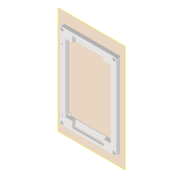
# Autodesk Inventor part: 30_xystage_gp-010b_adapter_multiwellplate
Saved by Autodesk Inventor 2022 (Build 260153000, 153)
## iProperties
Created: 2023-06-03
Part Number: 30_xystage_gp-010b_adapter_multiwellplate
Material: Generisch
Document SubType Name: Modeling
Designer: diederichbenedict
Density: 1 g/cm^3
Appearance: Vorgabe
Author: diederichbenedict
Autodesk Inventor part; units mm, degrees
ref_plane "YZ Plane" through (0, 0, 0) normal (1, 0, 0) x (0, 1, 0)
ref_plane "XZ Plane" through (0, 0, 0) normal (0, 1, 0) x (-1, 0, 0)
ref_plane "XY Plane" through (0, 0, 0) normal (0, 0, 1) x (1, 0, 0)
ref_plane "Arbeitsebene1" through (0, 0, 0) normal (0, 0, 1) x (1, 0, 0)
sketch "Skizze1" plane through (0, 0, 0) normal (0, 0, 1) x (1, 0, 0)
  line L0 (50, 77.5) -> (-50, 77.5) construction
  line L1 (-50, 77.5) -> (-50, -77.5) construction
  line L2 (-50, -77.5) -> (50, -77.5) construction
  line L3 (50, -77.5) -> (50, 77.5) construction
  line L4 (51, 82.5) -> (-51, 82.5)
  line L5 (-55, 78.5) -> (-55, -78.5)
  line L6 (-51, -82.5) -> (51, -82.5)
  line L7 (55, -78.5) -> (55, 78.5)
  circle A0 centre (50, 77.5) radius 1.6
  circle A1 centre (50, -77.5) radius 1.6
  circle A2 centre (-50, -77.5) radius 1.6
  circle A3 centre (-50, 77.5) radius 1.6
  arc A4 (55, 78.5) -> (51, 82.5) centre (51, 78.5) ccw
  arc A5 (51, -82.5) -> (55, -78.5) centre (51, -78.5) ccw
  arc A6 (-55, -78.5) -> (-51, -82.5) centre (-51, -78.5) ccw
  arc A7 (-51, 82.5) -> (-55, 78.5) centre (-51, 78.5) ccw
  line L8 (43, 64.5) -> (43, -64.5)
  line L9 (-43, -64.5) -> (-43, 64.5)
  line L10 (-43, 63.5) -> (-43, 64.5)
  line L11 (-43, 64.5) -> (43, 64.5)
  line L12 (43, 64.5) -> (43, 74.0537)
  line L13 (-43, -64.5) -> (43, -64.5)
  circle A8 centre (-43, 64.5) radius 5
  circle A9 centre (43, 64.5) radius 5
  circle A10 centre (43, -64.5) radius 5
  circle A11 centre (-43, -64.5) radius 5
  point P0 (0, 0)
  point P1 (-43, -59.5)
  point P2 (-43, 59.5)
  point P3 (-38, 64.5)
  point P4 (38, 64.5)
  point P5 (43, 59.5)
  point P6 (43, -59.5)
  point P7 (38, -64.5)
  point P8 (-38, -64.5)
  dimension "d1" = 3.2
  dimension "d2" = 3.2
  dimension "d3" = 3.2
  dimension "d4" = 3.2
  dimension "d5" = 4
  dimension "d6" = 86
  dimension "d10" = 10
  dimension "d11" = 10
  dimension "d12" = 10
  dimension "d13" = 10
  dimension "d31" = 43
  dimension "d32" = 129
  dimension "d33" = 100
  dimension "d34" = 155
  dimension "d35" = 64.5
  dimension "d36" = 55
  dimension "d37" = 110
  dimension "d38" = 165
  dimension "d39" = 82.5
  constraints: 28 end point, 12 centre point, 8 coincident, 8 point on circle, 8 tangent, 6 parallel, 3 equal radius, 2 perpendicular, 1 horizontal, 3 other
  measures "d1" diameter of A0
  measures "d2" diameter of A1
  measures "d3" diameter of A2
  measures "d4" diameter of A3
  measures "d5" radius of A4
  measures "d6" distance between parallel lines of L9 L8
  measures "d10" diameter of A8
  measures "d11" diameter of A9
  measures "d12" diameter of A10
  measures "d13" diameter of A11
  measures "d31" distance from line of point (0, 0) L8
  measures "d32" distance between parallel lines of L13 L11
  measures "d33" distance between parallel lines of L3 L1
  measures "d34" distance between parallel lines of L2 L0
  measures "d35" distance from line of point (0, 0) L11
  measures "d36" distance from line of L5 point (0, 0)
  measures "d37" distance between parallel lines of L7 L5
  measures "d38" distance between parallel lines of L6 L4
  measures "d39" distance from line of point (0, 0) L4
extrude "Extrusion1" add sketch "Skizze1" along normal blind 1 contours A4 L7 A5 L6 A6 L5 A7 L4 | L12 A9 L8 | L8 A9 L11 | L11 A9 L12 | A10 L13 L8 | L8 L13 A10 | A8 L9 L11 | L11 L9 A8 | A11 L9 L13 | L13 L9 A11
sketch "Skizze2" plane through (0, 0, 1) normal (0, 0, 1) x (1, 0, 0)
  arc A0 (-51, 82.5) -> (-55, 78.5) centre (-51, 78.5) ccw projected
  line L0 (-55, 78.5) -> (-55, -78.5) projected
  arc A1 (-55, -78.5) -> (-51, -82.5) centre (-51, -78.5) ccw projected
  line L1 (-51, -82.5) -> (51, -82.5) projected
  arc A2 (51, -82.5) -> (55, -78.5) centre (51, -78.5) ccw projected
  line L2 (55, -78.5) -> (55, 78.5) projected
  arc A3 (55, 78.5) -> (51, 82.5) centre (51, 78.5) ccw projected
  line L3 (51, 82.5) -> (-51, 82.5) projected
  arc A4 (-38, -64.5) -> (-43, -59.5) centre (-43, -64.5) ccw projected
  line L4 (-43, -59.5) -> (-43, 59.5) projected
  arc A5 (-43, 59.5) -> (-38, 64.5) centre (-43, 64.5) ccw projected
  line L5 (-38, 64.5) -> (38, 64.5) projected
  arc A6 (38, 64.5) -> (43, 59.5) centre (43, 64.5) ccw projected
  line L6 (43, 59.5) -> (43, -59.5) projected
  arc A7 (43, -59.5) -> (38, -64.5) centre (43, -64.5) ccw projected
  line L7 (38, -64.5) -> (-38, -64.5) projected
  circle A8 centre (-50, 77.5) radius 1.6 projected
  circle A9 centre (-50, -77.5) radius 1.6 projected
  circle A10 centre (50, -77.5) radius 1.6 projected
  circle A11 centre (50, 77.5) radius 1.6 projected
  line L8 (-43, 64.5) -> (43, 64.5)
  line L9 (43, 64.5) -> (43, -64.5)
  line L10 (43, -64.5) -> (-43, -64.5)
  line L11 (-43, -64.5) -> (-43, 64.5)
  point P0 (-43, 59.5)
  point P1 (43, -59.5)
  point P2 (38, -64.5)
  point P3 (-43, -59.5)
  constraints: 8 end point, 2 parallel, 1 horizontal, 1 perpendicular
extrude "Extrusion2" add sketch "Skizze2" along normal blind 6 draft -5
sketch "Skizze3" plane through (0, 0, 7) normal (0, 0, 1) x (1, 0, 0)
  line L0 (-44.539, -64.7031) -> (-50.539, -68.1672)
  line L1 (-50.539, -68.1672) -> (-50.539, -61.239)
  line L2 (-50.539, -61.239) -> (-44.539, -64.7031)
  line L3 (39.5249, 74.6999) -> (39.5249, -55.3499) projected
  point P0 (0, 0)
  point P1 (-48.539, -64.7031)
  dimension "d23" = 6
  constraints: 6 end point, 7 other
  measures "d23" distance from line of L1 L0.start
extrude "Extrusion3" cut sketch "Skizze3" against normal blind 1
sketch "Skizze4" plane through (0, 0, 7) normal (0, 0, 1) x (1, 0, 0)
  line L0 (-44.539, -64.7031) -> (-50.539, -68.1672) projected
  line L1 (-50.539, -61.239) -> (-44.539, -64.7031) projected
  circle A0 centre (-50, 77.5) radius 2.1249 projected
  circle A1 centre (-50, -77.5) radius 2.1249 projected
  circle A2 centre (50, -77.5) radius 2.1249 projected
  circle A3 centre (50, 77.5) radius 2.1249 projected
  line L2 (-54.4751, -78.5) -> (-54.4751, 78.5) projected
  arc A4 (-54.4751, -78.5) -> (-51, -81.9751) centre (-51, -78.5) ccw projected
  line L3 (51, -81.9751) -> (-51, -81.9751) projected
  arc A5 (51, -81.9751) -> (54.4751, -78.5) centre (51, -78.5) ccw projected
  line L4 (54.4751, 78.5) -> (54.4751, -78.5) projected
  arc A6 (54.4751, 78.5) -> (51, 81.9751) centre (51, 78.5) ccw projected
  line L5 (-51, 81.9751) -> (51, 81.9751) projected
  arc A7 (-51, 81.9751) -> (-54.4751, 78.5) centre (-51, 78.5) ccw projected
  circle A8 centre (-50, -77.5) radius 1.6 projected
  circle A9 centre (50, -77.5) radius 1.6 projected
  circle A10 centre (50, 77.5) radius 1.6 projected
  circle A11 centre (-50, 77.5) radius 1.6 projected
  line L6 (-50.539, -68.1672) -> (-50.539, -61.239) projected
  point P0 (0, 0)
  constraints: 4 coincident
hole "Bohrung1" at (-50, -77.5, 7) at (50, -77.5, 7) at (50, 77.5, 7) at (-50, 77.5, 7) direction (0, 0, -1) diameter 3.2 end through all counterbore diameter 6.5 counterbore depth 3
sketch "Skizze5" plane through (0, 0, 0) normal (1, 0, 0) x (0, 1, 0)
  line L0 (64.5, 1) -> (65.0249, 7) projected
  line L1 (64.5, 1) -> (71.5, 1)
  line L2 (76.5, 6) -> (76.5, 16)
  line L3 (76.5, 16) -> (64.5, 16)
  line L4 (64.5, 16) -> (64.5, 1)
  line L5 (-64.5, 0) -> (-64.5, 1) projected
  line L6 (-64.5, 1) -> (-71.5, 1)
  line L7 (-76.5, 6) -> (-76.5, 12.183)
  line L8 (-76.5, 12.183) -> (-64.5, 12.183)
  line L9 (-64.5, 12.183) -> (-64.5, 1)
  arc A0 (-76.5, 6) -> (-71.5, 1) centre (-71.5, 6) ccw
  arc A1 (71.5, 1) -> (76.5, 6) centre (71.5, 6) ccw
  point P0 (0, 0)
  point P1 (76.5, 1)
  dimension "d40" = 12
  dimension "d41" = 15
  dimension "d42" = 12
  dimension "d43" = 5
  constraints: 16 end point, 4 parallel, 4 point on circle, 4 tangent, 2 centre point, 2 horizontal, 2 perpendicular, 2 point on line, 1 equal radius
  measures "d40" distance of L3.end L2.end
  measures "d41" distance of L2.end point (76.5, 1)
  measures "d42" distance of L7.end L8.end
  measures "d43" radius of A0
extrude "Extrusion4" cut sketch "Skizze5" along normal mid plane 60
sketch "Skizze6" plane through (0, 0, 7) normal (0, 0, 1) x (1, 0, 0)
  circle A0 centre (-50, 77.5) radius 1.8625 projected
  line L0 (-43.5249, -65.0249) -> (-43.5249, 65.0249) projected
  line L1 (-43.5249, 65.0249) -> (-37.8681, 65.0249) construction
  circle A1 centre (-50, 52.5) radius 1.4
  point P0 (0, 0)
  dimension "d48" = 2.8
  dimension "d51" = 25
  constraints: 2 end point, 1 centre point, 1 horizontal
  measures "d48" diameter of A1
  measures "d51" distance of A1.centre A0.centre
extrude "Extrusion5" cut sketch "Skizze6" against normal blind 60 contours A1
sketch "Skizze7" plane through (0, 0, 7) normal (0, 0, 1) x (1, 0, 0)
  circle A0 centre (-50, 52.5) radius 1.4 projected
  line L0 (-54.4751, -78.5) -> (-54.4751, 78.5) projected
  arc A1 (-54.4751, -78.5) -> (-51, -81.9751) centre (-51, -78.5) ccw projected
  line L1 (51, -81.9751) -> (-51, -81.9751) projected
  arc A2 (51, -81.9751) -> (54.4751, -78.5) centre (51, -78.5) ccw projected
  line L2 (54.4751, 78.5) -> (54.4751, -78.5) projected
  arc A3 (54.4751, 78.5) -> (51, 81.9751) centre (51, 78.5) ccw projected
  line L3 (-51, 81.9751) -> (51, 81.9751) projected
  arc A4 (-51, 81.9751) -> (-54.4751, 78.5) centre (-51, 78.5) ccw projected
  line L4 (-44.539, -64.7031) -> (-50.539, -68.1672) projected
  line L5 (-50.539, -68.1672) -> (-50.539, -61.239) projected
  line L6 (-50.539, -61.239) -> (-44.539, -64.7031) projected
  circle A5 centre (-50, 77.5) radius 3.25 projected
  circle A6 centre (50, -77.5) radius 3.25 projected
  circle A7 centre (-50, -77.5) radius 3.25 projected
  circle A8 centre (50, 77.5) radius 3.25 projected
  line L7 (30, -65.0249) -> (30, -76.5) projected
  line L8 (30, -76.5) -> (-30, -76.5) projected
  line L9 (-30, -76.5) -> (-30, -65.0249) projected
  line L10 (-30, -65.0249) -> (-43.5249, -65.0249) projected
  line L11 (-43.5249, -65.0249) -> (-43.5249, 65.0249) projected
  line L12 (-43.5249, 65.0249) -> (-30, 65.0249) projected
  line L13 (-30, 65.0249) -> (-30, 76.5) projected
  line L14 (-30, 76.5) -> (30, 76.5) projected
  line L15 (30, 76.5) -> (30, 65.0249) projected
  line L16 (30, 65.0249) -> (43.5249, 65.0249) projected
  line L17 (43.5249, 65.0249) -> (43.5249, -65.0249) projected
  line L18 (43.5249, -65.0249) -> (30, -65.0249) projected
  line L19 (-50, -81.5) -> (50, -81.5)
  line L20 (54, -77.5) -> (54, 77.5)
  line L21 (50, 81.5) -> (-50, 81.5)
  line L22 (-54, 77.5) -> (-54, -77.5)
  line L23 (-54, -81.5) -> (54, 81.5) construction
  line L24 (54, -81.5) -> (-54, 81.5) construction
  arc A9 (54, 77.5) -> (50, 81.5) centre (50, 77.5) ccw
  arc A10 (-50, 81.5) -> (-54, 77.5) centre (-50, 77.5) ccw
  arc A11 (-54, -77.5) -> (-50, -81.5) centre (-50, -77.5) ccw
  arc A12 (50, -81.5) -> (54, -77.5) centre (50, -77.5) ccw
  point P0 (0, 0)
  dimension "d52" = 108
  dimension "d53" = 163
  dimension "d54" = 4
  constraints: 12 end point, 8 point on circle, 8 point on line, 8 tangent, 4 centre point, 3 equal radius, 2 midpoint, 2 parallel, 1 horizontal, 1 perpendicular
  measures "d52" distance of L24.end L23.end
  measures "d53" distance of L23.end L24.start
  measures "d54" radius of A9
extrude "Extrusion6" cut sketch "Skizze7" against normal blind 10 contours A0 | L0 A4 L3 A3 L2 A2 L1 A1 | L4 L5 L6 | A5 | A6 | A7 | A8 | L7 L8 L9 L10 L11 L12 L13 L14 L15 L16 L17 L18 | A11 L22 A10 L21 A9 L20 A12 L19 keep common part
equation "\"d11\" = d10"
equation "\"d12\" = d10"
equation "\"d13\" = d10"
equation "\"d31\" = 0.5 * d6"
equation "\"d35\" = 0.5 * d32"
equation "\"d36\" = 0.5 * d37"
equation "\"d39\" = 0.5 * d38"
